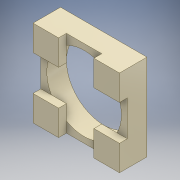
# Autodesk Inventor part: final cela
Saved by Autodesk Inventor 2017 (Build 210142000, 142)
## iProperties
Created: 2019-05-07
Part Number: final cela
Material: Tworzywo sztuczne ABS
Document SubType Name: Modeling
Designer: patry
Density: 1.06 g/cm^3
Appearance: Jasnobeżowa
Author: patry
Autodesk Inventor part; units mm, degrees
ref_plane "YZ Plane" through (0, 0, 0) normal (1, 0, 0) x (0, 1, 0)
ref_plane "XZ Plane" through (0, 0, 0) normal (0, 1, 0) x (-1, 0, 0)
ref_plane "XY Plane" through (0, 0, 0) normal (0, 0, 1) x (1, 0, 0)
sketch "Szkic1" plane through (0, 0, 0) normal (0, 1, 0) x (-1, 0, 0)
  circle A0 centre (0, 0) radius 9.5
  line L0 (-11, 11) -> (11, 11)
  line L1 (11, 11) -> (11, -11)
  line L2 (11, -11) -> (-11, -11)
  line L3 (-11, -11) -> (-11, 11)
  line L4 (-11, 11) -> (11, -11) construction
  line L5 (11, 11) -> (-11, -11) construction
  dimension "d0" = 19
  dimension "d1" = 22
  dimension "d2" = 22
  constraints: 12 end point, 2 midpoint, 2 parallel, 1 centre point, 1 coincident, 1 horizontal, 1 perpendicular
  measures "d0" diameter of A0
  measures "d1" distance of L1.end L2.end
  measures "d2" distance of L0.end L1.end
sketch "Szkic2" plane through (0, 0, 0) normal (0, 1, 0) x (-1, 0, 0)
  line L0 (11, -11) -> (-11, -11) projected
  line L1 (11, 11) -> (11, -11) projected
  line L2 (-11, 11) -> (11, 11) projected
  line L3 (-11, -11) -> (-11, 11) projected
  circle A0 centre (0, 0) radius 9.5 projected
  line L4 (11, -11) -> (4.5, -11)
  line L5 (4.5, -11) -> (4.5, -4.5)
  line L6 (4.5, -4.5) -> (11, -4.5)
  line L7 (11, -4.5) -> (11, -11)
  line L8 (-11, -11) -> (-4.5, -11)
  line L9 (-4.5, -11) -> (-4.5, -4.5)
  line L10 (-4.5, -4.5) -> (-11, -4.5)
  line L11 (-11, -4.5) -> (-11, -11)
  line L12 (-11, 11) -> (-4.5, 11)
  line L13 (-4.5, 11) -> (-4.5, 4.5)
  line L14 (-4.5, 4.5) -> (-11, 4.5)
  line L15 (-11, 4.5) -> (-11, 11)
  line L16 (11, 11) -> (4.5, 11)
  line L17 (4.5, 11) -> (4.5, 4.5)
  line L18 (4.5, 4.5) -> (11, 4.5)
  line L19 (11, 4.5) -> (11, 11)
  dimension "d3" = 6.5
  dimension "d4" = 6.5
  dimension "d5" = 6.5
  dimension "d6" = 6.5
  dimension "d7" = 6.5
  dimension "d8" = 6.5
  dimension "d9" = 6.5
  dimension "d10" = 6.5
  constraints: 32 end point, 8 parallel, 4 horizontal, 4 perpendicular
  measures "d3" distance of L5.end L6.end
  measures "d4" distance of L4.end L5.end
  measures "d5" distance of L10.end L9.end
  measures "d6" distance of L9.end L8.end
  measures "d7" distance of L13.end L14.end
  measures "d8" distance of L12.end L13.end
  measures "d9" distance of L18.end L17.end
  measures "d10" distance of L17.end L16.end
extrude "Wyciągnięcie proste1" add sketch "Szkic1" along normal blind 5
extrude "Wyciągnięcie proste2" add sketch "Szkic2" against normal blind 2 contours L0 L5 A0 L6 L1 | L0 L3 L10 A0 L9 | L5 L6 A0 | L18 A0 L17 L2 L1 | A0 L10 L9 | L18 L17 A0 | L3 L2 L13 A0 L14 | A0 L13 L14
equation "\"d3\" = d8"
equation "\"d4\" = d8"
equation "\"d5\" = d8"
equation "\"d6\" = d8"
equation "\"d7\" = d8"
equation "\"d9\" = d8"
equation "\"d10\" = d8"
